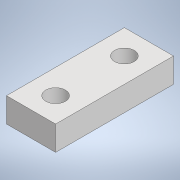
# Autodesk Inventor part: Metal_Bushing
Saved by Autodesk Inventor 2022 (Build 260153070, 153G)
## iProperties
Created: 2022-03-06
Part Number: Metal_Bushing
Material: Generic
Document SubType Name: Modeling
Designer: a laptop
Density: 1 g/cm^3
Appearance: Default
Author: a laptop
Autodesk Inventor part; units mm, degrees
ref_plane "YZ Plane" through (0, 0, 0) normal (1, 0, 0) x (0, 1, 0)
ref_plane "XZ Plane" through (0, 0, 0) normal (0, 1, 0) x (-1, 0, 0)
ref_plane "XY Plane" through (0, 0, 0) normal (0, 0, 1) x (1, 0, 0)
sketch "Sketch1" plane through (0, 0, 0) normal (0, 1, 0) x (-1, 0, 0)
  circle A0 centre (0, 7) radius 2
  circle A1 centre (0, -7) radius 2
  line L0 (0, 7) -> (0, -7)
  line L1 (5, -12) -> (-5, -12)
  line L2 (-5, -12) -> (-5, 12)
  line L3 (-5, 12) -> (5, 12)
  line L4 (5, 12) -> (5, -12)
  point P0 (0, 0)
  point P1 (0, 0)
  point P2 (-5, 0)
  point P3 (0, -12)
  dimension "d0" = 4
  dimension "d1" = 4
  dimension "d2" = 14
  dimension "d3" = 10
  dimension "d4" = 24
  constraints: 10 end point, 3 midpoint, 2 centre point, 2 parallel, 1 coincident, 1 horizontal, 1 horizontal alignment, 1 perpendicular, 1 vertical, 1 vertical alignment
  measures "d0" diameter of A1
  measures "d1" diameter of A0
  measures "d2" distance of L0.start L0.end
  measures "d3" distance of L1.start L1.end
  measures "d4" distance of L3.end L1.start
extrude "Extrusion1" add sketch "Sketch1" along normal blind 5
sketch "Sketch2" plane through (5, 0, -12) normal (0, 0, -1) x (-1, 0, 0)
  circle A0 centre (5, -5) radius 6
  circle A1 centre (5, -5) radius 3
  line L0 (0, 0) -> (0, 5) projected
  line L1 (10, 0) -> (0, 0) projected
  line L2 (0, 0) -> (0, -1.6834)
  line L3 (10, 0) -> (10, -1.6834)
  line L4 (2, -10.1962) -> (8, -10.1962)
  point P0 (5, 0)
  dimension "d7" = 6
  dimension "d8" = 5
  dimension "d9" = 5
  dimension "d10" = 12
  dimension "d11" = 6
  constraints: 6 end point, 4 point on circle, 2 centre point, 1 coincident, 1 horizontal, 1 parallel, 1 perpendicular
  measures "d7" diameter of A1
  measures "d8" distance of point (5, 0) A0.centre
  measures "d9" distance from line of L0 A0.centre
  measures "d10" diameter of A0
  measures "d11" distance of L4.start L4.end
extrude "Extrusion2" add sketch "Sketch2" against normal blind 24 contours A0 L4 L1 | A0 L1 L3 | A0 L2 L1
sketch "Sketch3" plane through (-3, -10.1962, -12) normal (0, -1, 0) x (1, 0, 0)
  circle A0 centre (3, 3) radius 1.5
  line L0 (3, 3) -> (3, 12) construction
  dimension "d14" = 3
  dimension "d15" = 9
  constraints: 2 end point, 1 centre point, 1 vertical
  measures "d14" diameter of A0
  measures "d15" distance of L0.start L0.end
extrude "Extrusion3" cut sketch "Sketch3" against normal blind 6.25
body "Solid1"
